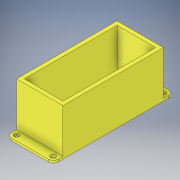
# Autodesk Inventor part: BatteryHolder
Saved by Autodesk Inventor 2018 (Build 220112000, 112)
## iProperties
Created: 2019-05-06
Part Number: BatteryHolder
Material: Generic
Document SubType Name: Modeling
Designer: jklei
Density: 1 g/cm^3
Appearance: Default
Author: jklei
Autodesk Inventor part; units mm, degrees
ref_plane "YZ Plane" through (0, 0, 0) normal (1, 0, 0) x (0, 1, 0)
ref_plane "XZ Plane" through (0, 0, 0) normal (0, 1, 0) x (-1, 0, 0)
ref_plane "XY Plane" through (0, 0, 0) normal (0, 0, 1) x (1, 0, 0)
sketch "Sketch1" plane through (0, 0, 0) normal (0, 1, 0) x (-1, 0, 0)
  line L0 (0, 0) -> (-31.75, 0)
  line L1 (-31.75, 0) -> (-31.75, -76.2)
  line L2 (-31.75, -76.2) -> (0, -76.2)
  line L3 (0, -76.2) -> (0, 0)
  line L4 (-34.925, -79.375) -> (-34.925, 3.175)
  line L5 (-34.925, 3.175) -> (3.175, 3.175)
  line L6 (3.175, 3.175) -> (3.175, -79.375)
  line L7 (3.175, -79.375) -> (-34.925, -79.375)
  dimension "d0" = 31.75
  dimension "d1" = 76.2
  dimension "d2" = 3.175
  constraints: 16 end point, 4 parallel, 2 perpendicular, 1 horizontal, 3 other
  measures "d0" distance of L2.end L1.end
  measures "d1" distance of L1.end L0.end
  measures "d2" distance between parallel lines of L1 L4
extrude "Extrusion1" add sketch "Sketch1" along normal blind 38.1
sketch "Sketch2" plane through (-3.175, 0, 3.175) normal (0, 0, 1) x (1, 0, 0)
  line L0 (38.1, 0) -> (38.1, 38.1) projected
  line L1 (0, 0) -> (38.1, 0)
  line L2 (38.1, 0) -> (38.1, 2)
  line L3 (38.1, 2) -> (0, 2)
  line L4 (0, 2) -> (0, 0)
  point P0 (3.175, 0)
  dimension "d5" = 2
  constraints: 8 end point, 2 parallel, 1 horizontal, 1 perpendicular, 1 point on line
  measures "d5" distance of L2.end L1.end
extrude "Extrusion2" add sketch "Sketch2" along normal blind 8
fillet "Fillet1" radius 4 2 edges at (34.925, 1, 11.175) (-3.175, 1, 11.175)
sketch "Sketch3" plane through (-3.175, 2, 3.175) normal (0, 1, 0) x (1, 0, 0)
  arc A0 (0, -4) -> (4, -8) centre (4, -4) ccw projected
  circle A1 centre (4, -4) radius 2.1
  arc A2 (34.1, -8) -> (38.1, -4) centre (34.1, -4) ccw projected
  circle A3 centre (34.1, -4) radius 2.1
  point P0 (3.175, 3.175)
  dimension "d9" = 4.2
  dimension "d10" = 4.2
  constraints: 2 centre point, 2 coincident
  measures "d9" diameter of A1
  measures "d10" diameter of A3
extrude "Extrusion3" cut sketch "Sketch3" against normal blind 8
sketch "Sketch4" plane through (34.925, 0, -79.375) normal (0, 0, -1) x (-1, 0, 0)
  line L0 (38.1, 2) -> (38.1, 0) projected
  line L1 (0, 0) -> (38.1, 0)
  line L2 (38.1, 0) -> (38.1, 2)
  line L3 (38.1, 2) -> (0, 2)
  line L4 (0, 2) -> (0, 0)
  point P0 (34.925, 0)
  dimension "d13" = 2
  constraints: 8 end point, 2 parallel, 1 horizontal, 1 perpendicular
  measures "d13" distance of L0.start L1.end
extrude "Extrusion4" add sketch "Sketch4" along normal blind 8
fillet "Fillet2" radius 4 2 edges at (34.925, 1, -87.375) (-3.175, 1, -87.375)
sketch "Sketch5" plane through (-3.175, 2, -79.375) normal (0, 1, 0) x (1, 0, 0)
  arc A0 (38.1, 4) -> (34.1, 8) centre (34.1, 4) ccw projected
  circle A1 centre (34.1, 4) radius 2.1
  arc A2 (4, 8) -> (0, 4) centre (4, 4) ccw projected
  circle A3 centre (4, 4) radius 2.1
  line L0 (4, 4) -> (0, 4)
  point P0 (3.175, -79.375)
  dimension "d17" = 4.2
  dimension "d18" = 4.2
  constraints: 2 centre point, 2 coincident, 2 end point, 1 horizontal
  measures "d17" diameter of A1
  measures "d18" diameter of A3
extrude "Extrusion5" cut sketch "Sketch5" against normal blind 8
body "Solid1"
